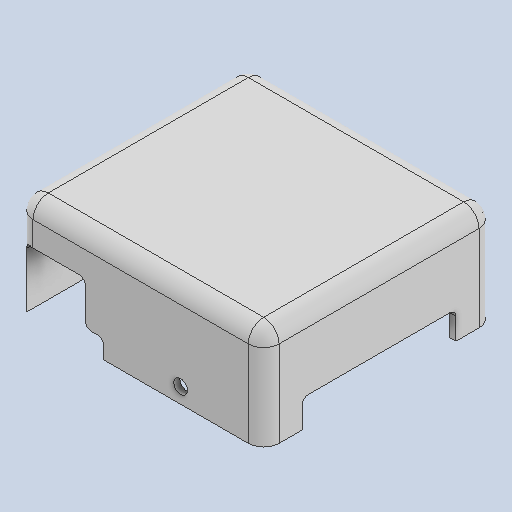
# Autodesk Inventor part: cable_box
Saved by Autodesk Inventor 2025 (Build 290162000, 162)
## iProperties
Created: 2025-09-20
Part Number: cable_box
Material: Generic
Document SubType Name: Modeling
Designer: Pravoslav
Density: 1 g/cm^3
Appearance: Default
Author: Pravoslav
Autodesk Inventor part; units mm, degrees
ref_plane "YZ Plane" through (0, 0, 0) normal (1, 0, 0) x (0, 1, 0)
ref_plane "XZ Plane" through (0, 0, 0) normal (0, 1, 0) x (-1, 0, 0)
ref_plane "XY Plane" through (0, 0, 0) normal (0, 0, 1) x (1, 0, 0)
sketch "Sketch1" plane through (0, 0, 0) normal (0, 1, 0) x (-1, 0, 0)
  line L0 (40, 37.5) -> (-40, 37.5)
  line L1 (-40, 37.5) -> (-40, -37.5)
  line L2 (-40, -37.5) -> (40, -37.5)
  line L3 (40, -37.5) -> (40, 37.5)
  line L4 (40, 37.5) -> (-40, -37.5) construction
  line L5 (-40, 37.5) -> (40, -37.5) construction
  point P0 (0, 0)
  dimension "d0" = 80
  dimension "d1" = 75
  constraints: 12 end point, 2 midpoint, 2 parallel, 1 horizontal, 1 perpendicular
  measures "d0" distance of L2.end L1.end
  measures "d1" distance of L1.end L0.end
extrude "Extrusion1" add sketch "Sketch1" along normal blind 3
sketch "Sketch2" plane through (0, 0, 0) normal (0, -1, 0) x (1, 0, 0)
  line L0 (-38, -35.5) -> (38, -35.5)
  line L1 (38, -35.5) -> (38, 35.5)
  line L2 (38, 35.5) -> (-38, 35.5)
  line L3 (-38, 35.5) -> (-38, -35.5)
  line L4 (-38, -35.5) -> (38, 35.5) construction
  line L5 (38, -35.5) -> (-38, 35.5) construction
  line L6 (-40, -37.5) -> (-40, 37.5) projected
  line L7 (-40, 37.5) -> (40, 37.5) projected
  line L8 (-40, -37.5) -> (40, -37.5)
  line L9 (40, -37.5) -> (40, 37.5)
  line L10 (40, 37.5) -> (-40, 37.5)
  line L11 (-40, 37.5) -> (-40, -37.5)
  line L12 (-40, -37.5) -> (40, 37.5) construction
  line L13 (40, -37.5) -> (-40, 37.5) construction
  point P0 (0, 0)
  dimension "d4" = 2
  dimension "d5" = 2
  constraints: 24 end point, 4 midpoint, 4 parallel, 2 horizontal, 2 perpendicular
  measures "d4" distance between parallel lines of L6 L3
  measures "d5" distance between parallel lines of L7 L2
extrude "Extrusion2" add sketch "Sketch2" along normal blind 30
sketch "Sketch3" plane through (40, 3, 37.5) normal (1, 0, 0) x (0, 0, -1)
  line L0 (73, -33) -> (2, -33) projected
  line L1 (12.5, -33) -> (62.5, -33)
  line L2 (62.5, -33) -> (62.5, -24)
  line L3 (62.5, -24) -> (12.5, -24)
  line L4 (12.5, -24) -> (12.5, -33)
  line L5 (75, -33) -> (75, 0) projected
  point P0 (37.5, -3)
  dimension "d8" = 50
  dimension "d9" = 9
  dimension "d10" = 12.5
  constraints: 8 end point, 2 parallel, 1 horizontal, 1 perpendicular, 1 point on line
  measures "d8" distance between parallel lines of L2 L4
  measures "d9" distance between parallel lines of L0 L3
  measures "d10" distance between parallel lines of L5 L2
extrude "Extrusion3" cut sketch "Sketch3" against normal up to surface (2 mm away)
sketch "Sketch4" plane through (-40, 3, 37.5) normal (0, 0, 1) x (1, 0, 0)
  line L0 (78, -33) -> (2, -33) projected
  line L1 (2, -33) -> (22, -33)
  line L2 (22, -33) -> (22, -13)
  line L3 (22, -13) -> (2, -13)
  line L4 (2, -13) -> (2, -33)
  line L5 (0, -33) -> (0, 0) projected
  line L6 (22, -33) -> (28, -33)
  line L7 (28, -33) -> (28, -27)
  line L8 (28, -27) -> (22, -27)
  line L9 (22, -27) -> (22, -33)
  point P0 (40, -3)
  point P1 (22, -27)
  dimension "d13" = 20
  dimension "d14" = 20
  dimension "d15" = 2
  dimension "d16" = 6
  dimension "d17" = 6
  constraints: 16 end point, 4 parallel, 2 horizontal, 2 perpendicular, 1 point on line
  measures "d13" distance between parallel lines of L2 L4
  measures "d14" distance between parallel lines of L0 L3
  measures "d15" distance between parallel lines of L5 L4
  measures "d16" distance of L8.end L7.end
  measures "d17" distance of L7.end L6.end
extrude "Extrusion4" cut sketch "Sketch4" against normal up to surface (2 mm away)
fillet "Fillet1" radius 2 4 edges at (-38, -10, 36.5) (-18, -10, 36.5) (-12, -24, 36.5) (-18, -24, 36.5)
fillet "Fillet2" radius 2 2 edges at (39, -21, 25) (39, -21, -25)
sketch "Sketch5" plane through (40, 3, -37.5) normal (0, 0, -1) x (-1, 0, 0)
  line L0 (2, -33) -> (78, -33) projected
  line L1 (78, -33) -> (63, -33)
  line L2 (63, -33) -> (63, -23)
  line L3 (63, -23) -> (78, -23)
  line L4 (78, -23) -> (78, -33)
  line L5 (80, -33) -> (80, 0) projected
  point P0 (40, -3)
  point P1 (78, -28)
  dimension "d22" = 15
  dimension "d23" = 10
  dimension "d24" = 2
  constraints: 8 end point, 2 parallel, 1 horizontal, 1 midpoint, 1 perpendicular, 1 point on line
  measures "d22" distance from line of point (78, -28) L2
  measures "d23" distance between parallel lines of L0 L3
  measures "d24" distance between parallel lines of L5 L4
extrude "Extrusion5" cut sketch "Sketch5" against normal up to surface (2 mm away)
fillet "Fillet3" radius 2 3 edges at (-38, -20, -36.5) (-23, -20, -36.5) (-23, -30, -36.5)
sketch "Sketch6" plane through (40, 3, -37.5) normal (0, 0, -1) x (-1, 0, 0)
  circle A0 centre (27, -28) radius 2.25
  line L0 (61, -33) -> (0, -33) projected
  line L1 (0, -33) -> (0, 0) projected
  point P0 (40, -3)
  dimension "d28" = 4.5
  dimension "d29" = 5
  dimension "d30" = 27
  constraints: 1 centre point
  measures "d28" diameter of A0
  measures "d29" distance from line of L0 A0.centre
  measures "d30" distance from line of L1 A0.centre
extrude "Extrusion6" cut sketch "Sketch6" against normal through all
sketch "Sketch7" plane through (-40, 3, -37.5) normal (-1, 0, 0) x (0, 0, 1)
  circle A0 centre (37.5, -28) radius 2.25
  line L0 (75, -33) -> (0, -33) projected
  line L1 (75, -33) -> (75, 0) projected
  point P0 (37.5, -3)
  dimension "d33" = 4.5
  dimension "d34" = 5
  dimension "d35" = 37.5
  constraints: 1 centre point
  measures "d33" diameter of A0
  measures "d34" distance from line of L0 A0.centre
  measures "d35" distance from line of L1 A0.centre
extrude "Extrusion7" cut sketch "Sketch7" against normal up to surface (2 mm away)
fillet "Fillet4" radius 5 4 edges at (-40, 3, 0) (0, 3, 37.5) (0, 3, -37.5) (40, 3, 0)
fillet "Fillet5" radius 5 8 edges at (38.5355, 1.5355, -36.0355) (40, -16, -37.5) (-38.5355, 1.5355, -36.0355) (-40, -16, -37.5) (-38.5355, 1.5355, 36.0355) (-40, -16, 37.5) (38.5355, 1.5355, 36.0355) (40, -16, 37.5)
body "Solid1"
